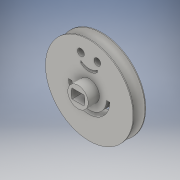
# Autodesk Inventor part: Wheel
Saved by Autodesk Inventor 2016 (Build 200138000, 138)
## iProperties
Created: 2017-09-08
Part Number: Wheel
Material: Generic
Document SubType Name: Modeling
Designer: student
Density: 1 g/cm^3
Appearance: Default
Author: student
Autodesk Inventor part; units mm, degrees
ref_plane "YZ Plane" through (0, 0, 0) normal (1, 0, 0) x (0, 1, 0)
ref_plane "XZ Plane" through (0, 0, 0) normal (0, 1, 0) x (-1, 0, 0)
sketch "Sketch1" plane through (0, 0, 0) normal (0, 0, 1) x (1, 0, 0)
  circle A0 centre (0, 0) radius 21.717
  dimension "d0" = 43.434
  constraints: 1 centre point, 1 coincident
  measures "d0" diameter of A0
extrude "Extrusion1" add sketch "Sketch1" along normal blind 6.35
sketch "Sketch2" plane through (0, 0, 0) normal (1, 0, 0) x (0, 1, 0)
  line L0 (-21.717, 0) -> (-21.717, 6.35) projected
  circle A0 centre (-21.717, 3.175) radius 2.7305
  point P0 (0, 0)
  dimension "d3" = 5.461
  constraints: 1 centre point, 1 midpoint
  measures "d3" diameter of A0
ref_plane "Work Plane1" through (0, 0, 3.175) normal (0, 0, 1) x (1, 0, 0)
sketch "Sketch3" plane through (0, 0, 3.175) normal (0, 0, 1) x (1, 0, 0)
  circle A0 centre (0, 0) radius 21.717
  dimension "d4" = 43.434
  constraints: 1 centre point, 1 coincident
  measures "d4" diameter of A0
sweep "Sweep1" cut profiles "Sketch2" path "Sketch3"
sketch "Sketch4" plane through (0, 0, 6.35) normal (0, 0, 1) x (1, 0, 0)
  circle A0 centre (0, 0) radius 5.08
  line L0 (3.4671, -2.3876) -> (-3.4671, -2.3876)
  line L1 (-3.4671, -2.3876) -> (-3.4671, 2.3876)
  line L2 (-3.4671, 2.3876) -> (3.4671, 2.3876)
  line L3 (3.4671, 2.3876) -> (3.4671, -2.3876)
  line L4 (3.4671, -2.3876) -> (-3.4671, 2.3876) construction
  line L5 (-3.4671, -2.3876) -> (3.4671, 2.3876) construction
  dimension "d7" = 10.16
  dimension "d8" = 6.9342
  dimension "d9" = 4.7752
  constraints: 12 end point, 2 midpoint, 2 parallel, 1 centre point, 1 coincident, 1 horizontal, 1 perpendicular
  measures "d7" diameter of A0
  measures "d8" distance of L1.end L2.end
  measures "d9" distance of L0.end L1.end
extrude "Extrusion2" add sketch "Sketch4" along normal blind 5.588 contours A0 | L0 L1 L2 L3
sketch "Sketch5" plane through (0, 0, 6.35) normal (0, 0, 1) x (1, 0, 0)
  circle A0 centre (-4.1364, 14.2824) radius 1.7313
  circle A1 centre (4.031, 14.2824) radius 1.6864
  arc A2 (-4.1364, 9.6984) -> (4.031, 9.6907) centre (-0.0484, 14.1988) ccw
  arc A3 (-4.1364, 10.8081) -> (4.031, 10.8001) centre (-0.0479, 15.6642) ccw
  line L0 (-4.1364, 9.6984) -> (-4.1364, 10.8081)
  line L1 (4.031, 9.6907) -> (4.031, 10.8001)
  arc A4 (-8.5875, 0) -> (8.6512, 0) centre (0.0318, 0.2386) ccw
  arc A5 (-10.2672, 0) -> (10.1982, 0) centre (-0.0345, -0.0517) ccw
  line L2 (-10.2672, 0) -> (-8.5875, 0)
  line L3 (8.6512, 0) -> (10.1982, 0)
  point P0 (0, 0)
  constraints: 8 end point, 8 point on circle, 6 centre point, 1 collinear, 1 horizontal, 1 parallel, 1 vertical
extrude "Extrusion3" cut sketch "Sketch5" against normal blind 25.4
sketch "Sketch6" plane through (0, 0, 11.938) normal (0, 0, 1) x (1, 0, 0)
  line L0 (2.9579, -2.3876) -> (-2.9579, -2.3876)
  line L1 (-2.9579, 2.3876) -> (2.9579, 2.3876)
  arc A0 (-2.9579, 2.3876) -> (-2.9579, -2.3876) centre (2.3852, 0) ccw
  arc A1 (2.9579, -2.3876) -> (2.9579, 2.3876) centre (-2.3852, 0) ccw
  constraints: 4 end point, 4 point on circle, 2 centre point, 1 horizontal, 1 parallel
extrude "Extrusion4" cut sketch "Sketch6" against normal blind 5.588
body "Solid1"
